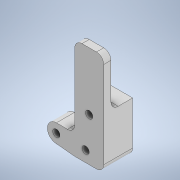
# Autodesk Inventor part: front_v2
Saved by Autodesk Inventor 2021 (Build 250183000, 183)
## iProperties
Created: 2025-12-28
Part Number: front_v2
Material: Generic
Document SubType Name: Modeling
Designer: Toby
Density: 1 g/cm^3
Appearance: Default
Author: Toby
Autodesk Inventor part; units mm, degrees
ref_plane "YZ Plane" through (0, 0, 0) normal (1, 0, 0) x (0, 1, 0)
ref_plane "XZ Plane" through (0, 0, 0) normal (0, 1, 0) x (-1, 0, 0)
ref_plane "XY Plane" through (0, 0, 0) normal (0, 0, 1) x (1, 0, 0)
sketch "Sketch1" plane through (0, 0, 0) normal (0, 0, 1) x (1, 0, 0)
  circle A0 centre (30, 0) radius 1
  circle A1 centre (21.926, 0) radius 1
  line L0 (27, 11) -> (35, 11)
  line L1 (35, 11) -> (35, -3)
  line L2 (35, -3) -> (27, -3)
  line L3 (27, -3) -> (27, 11)
  circle A2 centre (21.926, 0) radius 2.5
  line L4 (21.926, -2.5) -> (27, -3)
  line L5 (21.926, 2.5) -> (27, 2.5)
  point P0 (0, 0)
  dimension "d0" = 21.926
  dimension "d1" = 30
  dimension "d2" = 2
  dimension "d3" = 2
  dimension "d4" = 3
  dimension "d5" = 5
  dimension "d6" = 3
  dimension "d7" = 11
  dimension "d8" = 5
  constraints: 12 end point, 3 centre point, 3 coincident, 2 parallel, 2 perpendicular, 2 point on circle, 1 horizontal, 1 point on line, 1 tangent
  measures "d0" distance of point (0, 0) point (21.926, 0)
  measures "d1" distance of point (0, 0) point (30, 0)
  measures "d2" diameter of A0
  measures "d3" diameter of A1
  measures "d4" distance from line of L3 A0.centre
  measures "d5" distance from line of L1 A0.centre
  measures "d6" distance from line of L2 point (30, 0)
  measures "d7" distance from line of point (30, 0) L0
  measures "d8" diameter of A2
extrude "Extrusion1" add sketch "Sketch1" along normal blind 8
fillet "Fillet1" radius 2 2 edges at (27, 2.5, 4) (35, -3, 4)
sketch "Sketch2" plane through (0, 0, 8) normal (0, 0, 1) x (1, 0, 0)
  line L0 (27, 11) -> (27, 4.5) projected
  line L1 (27, 11) -> (35, 11)
  line L2 (35, 11) -> (35, 25)
  line L3 (35, 25) -> (27, 25)
  line L4 (27, 25) -> (27, 11)
  line L5 (35, -1) -> (35, 11) projected
  circle A0 centre (30, 0) radius 1 projected
  point P0 (0, 0)
  dimension "d12" = 25
  constraints: 8 end point, 2 parallel, 1 collinear, 1 horizontal, 1 perpendicular
  measures "d12" distance from line of A0.centre L3
extrude "Extrusion2" add sketch "Sketch2" against normal blind 2 contours L4 L3 L2 L1
fillet "Fillet2" radius 2 1 edges at (31, 11, 6)
fillet "Fillet3" radius 2 2 edges at (35, 25, 7) (27, 25, 7)
sketch "Sketch3" plane through (0, 0, 8) normal (0, 0, 1) x (1, 0, 0)
  line L0 (35, -1) -> (35, 23) projected
  line L1 (27, 23) -> (27, 4.5) projected
  circle A0 centre (30, 0) radius 1 projected
  point P0 (0, 0)
  point P1 (31, 9)
  dimension "d17" = 8
  dimension "d18" = 4
  dimension "d19" = 9
  measures "d17" distance between parallel lines of L0 L1
  measures "d18" distance from line of L1 point (31, 9)
  measures "d19" vertical distance of A0.centre point (31, 9)
hole "Hole1" at (31, 9, 8) direction (0, 0, -1) diameter 2 depth 5 tip angle 118
sketch "Sketch4" plane through (0, 0, 0) normal (0, 0, -1) x (-1, 0, 0)
  line L0 (-27, 11) -> (-27, 4.5) projected
  line L1 (-17, -3) -> (-27, -3)
  line L2 (-27, -3) -> (-27, 5)
  line L3 (-27, 5) -> (-17, 5)
  line L4 (-17, 5) -> (-17, -3)
  line L5 (-27, -3) -> (-33, -3) projected
  point P0 (0, 0)
  dimension "d27" = 10
  dimension "d28" = 8
  constraints: 8 end point, 2 parallel, 1 collinear, 1 horizontal, 1 perpendicular, 1 point on line
  measures "d27" distance of L2.end L3.end
  measures "d28" distance of L3.end L1.start
extrude "Extrusion3" cut sketch "Sketch4" against normal blind 3
fillet "Fillet4" radius 2 1 edges at (27, 0.75, 3)
body "Solid1"
